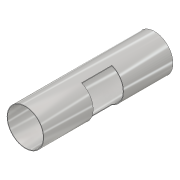
# Autodesk Inventor part: DPLX_P007_Wire_Mesh_Sleeve_Spark_Gap
Saved by Autodesk Inventor 2018 (Build 220112000, 112)
## iProperties
Created: 2018-06-06
Part Number: DPLX_P007_Wire_Mesh_Sleeve_Spark_Gap
Material: Stucco
Document SubType Name: Modeling
Designer: DPLXuser
Density: 1.9 g/cm^3
Appearance: Aluminum - Polished
Author: DPLXuser
Autodesk Inventor part; units mm, degrees
ref_plane "YZ Plane" through (0, 0, 0) normal (1, 0, 0) x (0, 1, 0)
ref_plane "XZ Plane" through (0, 0, 0) normal (0, 1, 0) x (-1, 0, 0)
ref_plane "XY Plane" through (0, 0, 0) normal (0, 0, 1) x (1, 0, 0)
sketch "Sketch1" plane through (0, 0, 0) normal (0, 1, 0) x (-1, 0, 0)
  circle A0 centre (0, 0) radius 15.175
  circle A1 centre (0, 0) radius 15.7084
  dimension "d1" = 30.35
  dimension "d2" = 31.4168
  constraints: 2 centre point, 2 coincident
  measures "d1" diameter of A0
  measures "d2" diameter of A1
extrude "Extrusion1" add sketch "Sketch1" along normal blind 110
sketch "Sketch3" plane through (0, 0, 0) normal (0, 0, 1) x (1, 0, 0)
  line L0 (15.7084, 42) -> (15.7084, 68)
  line L1 (15.7084, 68) -> (5.7084, 68)
  line L2 (5.7084, 68) -> (5.7084, 42)
  line L3 (15.7084, 42) -> (5.7084, 42)
  point P0 (0, 0)
  dimension "d7" = 26
  dimension "d8" = 10
  constraints: 8 end point, 2 perpendicular, 1 horizontal
  measures "d7" distance of L0.start L0.end
  measures "d8" distance of L0.end L1.end
extrude "Extrusion2" cut sketch "Sketch3" along normal mid plane 110
body "Solid1"
